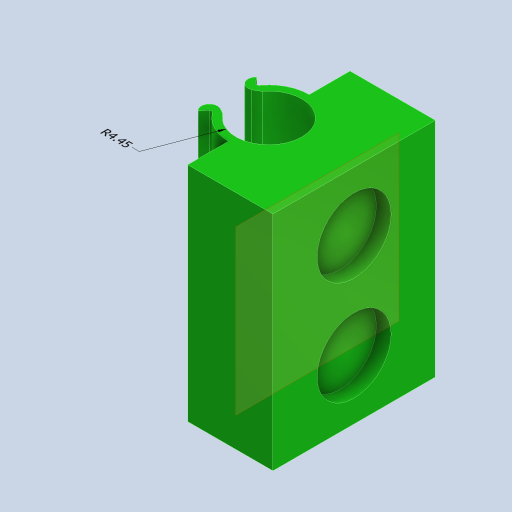
# Autodesk Inventor part: крепление маркера 9мм
Saved by Autodesk Inventor 2024.2 (Build 282272000, 272)
## iProperties
Created: 2025-12-12
Part Number: крепление маркера 9мм
Material: Типовые
Document SubType Name: Modeling
Designer: katya_notebook
Density: 1 g/cm^3
Appearance: Темно-зеленый
Author: katya_notebook
Autodesk Inventor part; units mm, degrees
ref_plane "YZ Plane" through (0, 0, 0) normal (1, 0, 0) x (0, 1, 0)
ref_plane "XZ Plane" through (0, 0, 0) normal (0, 1, 0) x (-1, 0, 0)
ref_plane "XY Plane" through (0, 0, 0) normal (0, 0, 1) x (1, 0, 0)
sketch "Эскиз1" plane through (0, 0, 0) normal (0, 1, 0) x (-1, 0, 0)
  circle A0 centre (0, 0) radius 4.45
  circle A1 centre (0, 0) radius 5.45
  line L0 (0, 0) -> (4.349, 3.2846)
  line L1 (0, 0) -> (4.349, -3.2846)
  point P0 (3.551, -2.6819)
  point P1 (3.551, 2.6819)
  dimension "d0" = 8.9
  dimension "d1" = 10.9
  constraints: 4 end point, 2 centre point, 2 coincident, 2 point on circle
  measures "d0" diameter of A0
  measures "d1" diameter of A1
extrude "Выдавливание1" add sketch "Эскиз1" along normal blind 30 contours A0 L1 A1 L0 picked at (-3.4029, -3.7722)
sketch "Эскиз2" plane through (0, 30, 0) normal (0, 1, 0) x (1, 0, 0)
  arc A0 (-3.551, -2.6819) -> (-4.4437, -2.1521) centre (-6.2523, -6.2159) ccw
  arc A1 (-4.4437, -2.1521) -> (-5.6006, -3.9578) centre (-4.878, -3.1473) ccw
  line L0 (-5.6006, -3.9578) -> (-4.9293, -3.1033)
  arc A2 (-4.3504, -3.2701) -> (-4.9293, -3.1033) centre (-4.7187, -3.4605) ccw
  line L1 (-3.551, -2.6819) -> (-4.349, -3.2846)
  line L2 (-4.349, -3.2846) -> (-3.551, -2.6819)
  line L3 (-4.349, -3.2846) -> (-4.3504, -3.2701)
  line L4 (-0.0151, 0) -> (-3.489, 0)
  arc A3 (-4.4437, 2.1521) -> (-3.551, 2.6819) centre (-6.2523, 6.2159) ccw
  arc A4 (-4.9293, 3.1033) -> (-4.3504, 3.2701) centre (-4.7187, 3.4605) ccw
  line L5 (-3.551, 2.6819) -> (-4.349, 3.2846)
  line L6 (-4.349, 3.2846) -> (-3.551, 2.6819)
  line L7 (-4.349, 3.2846) -> (-4.3504, 3.2701)
  arc A5 (-5.6006, 3.9578) -> (-4.4437, 2.1521) centre (-4.878, 3.1473) ccw
  line L8 (-5.6006, 3.9578) -> (-4.9293, 3.1033)
  point P0 (-3.551, 2.6819)
  point P1 (-4.349, -3.2846)
  point P2 (-5.3694, -4.0591)
  point P3 (-4.349, 3.2846)
  point P4 (-5.3694, 4.0591)
  point P5 (-4.349, 3.2846)
  dimension "d25" = 1.0859
  constraints: 18 end point, 12 point on circle, 12 symmetric about line, 6 centre point, 4 coincident, 1 collinear, 1 horizontal, 3 other
  measures "d25" radius of A1
sketch "Эскиз3" plane through (0, 30, 0) normal (0, 1, 0) x (1, 0, 0)
  arc A0 (-4.349, -3.2846) -> (-4.349, 3.2846) centre (0, 0) ccw projected
  line L0 (11.5, -6.95) -> (11.5, 6.95)
  arc A1 (-3.551, -2.6819) -> (-3.551, 2.6819) centre (0, 0) ccw projected
  line L1 (0, -5.45) -> (0, -4.45)
  line L2 (0, 4.45) -> (0, 5.45)
  line L3 (11.5, 6.95) -> (11.5, 10.95)
  line L4 (11.5, -6.95) -> (11.5, -10.95)
  line L5 (0, 0.95) -> (0, 5.45)
  line L6 (11.5, -10.95) -> (0, -10.95)
  line L7 (0, -10.95) -> (0, -5.45)
  line L8 (11.5, 10.95) -> (0, 10.95)
  line L9 (0, 10.95) -> (0, 5.45)
  arc A2 (0, -4.45) -> (0, 4.45) centre (0, 0) ccw
  dimension "d13" = 4
  dimension "d14" = 4
  dimension "d22" = 21.9
  dimension "d23" = 6.5
  constraints: 20 end point, 6 point on circle, 4 vertical, 2 horizontal, 2 perpendicular, 1 centre point, 1 collinear, 1 concentric
  measures "d13" distance of L4.end L0.start
  measures "d14" distance of L3.end L0.end
  measures "d22" distance of L4.end L3.end
  measures "d23" distance of L6.end L1.end
extrude "Выдавливание3" add sketch "Эскиз3" against normal blind 30
ref_plane "РабПлоскость1" through (11.5, 20, 4.95) normal (1, 0, 0) x (0, 0, -1)
sketch "Эскиз4" plane through (11.5, 20, 4.95) normal (1, 0, 0) x (0, 0, -1)
  line L0 (4.95, -20) -> (4.95, 10)
  line L1 (1, 10) -> (8.9, 10) projected
  circle A0 centre (4.95, -12) radius 5
  line L2 (14.4, -20) -> (-4.5, -20) projected
  circle A1 centre (4.95, 2) radius 5
  line L3 (-4.5, 10) -> (14.4, 10) projected
  point P0 (7.3306, 10)
  point P1 (2.5694, 10)
  point P2 (4.95, 10)
  dimension "d15" = 10
  dimension "d16" = 8
  dimension "d17" = 10
  dimension "d18" = 8
  constraints: 3 midpoint, 2 centre point, 2 end point, 2 point on line
  measures "d15" diameter of A0
  measures "d16" distance of A0.centre point (4.95, -20)
  measures "d17" diameter of A1
  measures "d18" distance of point (4.95, 10) A1.centre
extrude "Выдавливание4" cut sketch "Эскиз4" against normal blind 2
extrude "Выдавливание5" add sketch "Эскиз2" against normal blind 30
sketch "Эскиз5" plane through (0, 30, 0) normal (0, 1, 0) x (1, 0, 0)
  arc A0 (0, 5.45) -> (-4.349, 3.2846) centre (0, 0) ccw projected
  line L0 (-4.349, 3.2846) -> (-4.3504, 3.2701) projected
  arc A1 (-4.9293, 3.1033) -> (-4.3504, 3.2701) centre (-4.7187, 3.4605) ccw projected
  line L1 (-4.9293, 3.1033) -> (-5.6006, 3.9578) projected
  arc A2 (-5.6006, 3.9578) -> (-4.4437, 2.1521) centre (-4.878, 3.1473) ccw projected
  arc A3 (-4.4437, 2.1521) -> (-3.551, 2.6819) centre (-6.2523, 6.2159) ccw projected
  arc A4 (-3.551, -2.6819) -> (-3.551, 2.6819) centre (0, 0) ccw projected
  arc A5 (-3.551, -2.6819) -> (-4.4437, -2.1521) centre (-6.2523, -6.2159) ccw projected
  arc A6 (-4.4437, -2.1521) -> (-5.6006, -3.9578) centre (-4.878, -3.1473) ccw projected
  line L2 (-5.6006, -3.9578) -> (-4.9293, -3.1033) projected
  arc A7 (-4.3504, -3.2701) -> (-4.9293, -3.1033) centre (-4.7187, -3.4605) ccw projected
  line L3 (-4.3504, -3.2701) -> (-4.349, -3.2846) projected
  arc A8 (-4.349, -3.2846) -> (0, -5.45) centre (0, 0) ccw projected
  line L4 (0, -5.45) -> (0, -10.95) projected
  line L5 (0, -10.95) -> (11.5, -10.95) projected
  line L6 (11.5, -10.95) -> (11.5, 10.95) projected
  line L7 (11.5, 10.95) -> (0, 10.95) projected
  line L8 (0, 10.95) -> (0, 5.45) projected
  line L9 (0, 4.45) -> (0, 5.45)
  line L10 (0, -4.45) -> (0, -5.45)
  constraints: 4 end point, 2 point on circle, 1 collinear, 1 point on line, 1 vertical
extrude "Выдавливание6" [suppressed]
sketch "Эскиз6" plane through (11.5, 30, 10.95) normal (1, 0, 0) x (0, 0, -1)
  arc A0 (15.95, -22) -> (15.95, -22) centre (10.95, -22) ccw projected
  arc A1 (15.95, -8) -> (15.95, -8) centre (10.95, -8) ccw projected
  point P0 (10.95, -30)
extrude "Выдавливание7" [suppressed]
